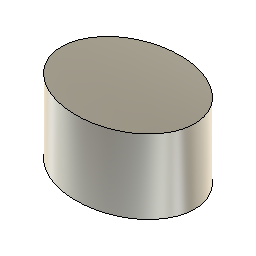
Seed Distribution System v19 (Autodesk Fusion 360 archive; units mm, degrees)
design "Maize Approximation"
Autodesk Fusion 360 part; units mm, degrees
note: some values were not read from the file. Set by a fixed rule: which face or edge a step refers to.
sketch "Sketch1" plane through (0, 0, 0) normal (0, 0, 1) x (1, 0, 0)
  ellipse E0 centre (0, 0) end of major axis (4.5, 0) minor radius 3.5
  line L0 (-4.5, 0) -> (4.5, 0) construction
  line L1 (0, -3.5) -> (0, 3.5) construction
  dimension "d1" = 7
  constraint coincident E0 L0.start
  constraint coincident E0 L0.end
  constraint coincident E0 L1.start
  constraint coincident E0 L1.end
  constraint coincident E0.centre origin
  constraint horizontal L0
extrude "Extrude1" add sketch "Sketch1" along normal blind 5

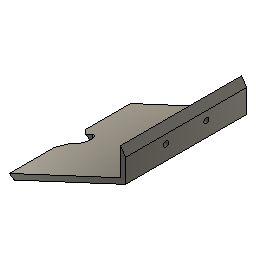
design "H-L1"
Autodesk Fusion 360 part; units mm, degrees
sketch "Sketch1" plane through (0, 0, 0) normal (0, 1, 0) x (1, 0, 0)
  line L0 (0, 0) -> (0, -20)
  line L1 (0, -20) -> (5, -20)
  line L2 (5, -20) -> (5, 0)
  line L3 (0, 0) -> (-107.5153, 50.1352)
  line L4 (-107.5153, 50.1352) -> (-105.4022, 54.6667)
  line L5 (5, 0) -> (5, 3.186)
  line L6 (-105.4022, 54.6667) -> (5, 3.1854)
  line L7 (0, -20) -> (0, -27.5)
  line L8 (0, -27.5) -> (5, -20)
  line L9 (-105.4022, 54.6667) -> (-110.1316, 51.3552)
  line L10 (-105.4022, 54.6667) -> (-105.6539, 54.6667) construction
  line L11 (-110.1316, 51.3552) -> (-107.5153, 50.1352)
  line L12 (0, 0) -> (0, 5.5169) construction
  dimension "d1" = 20
  dimension "d2" = 5
  dimension "d3" = 118.63
  dimension "d4" = 115
  dimension "d5" = 5
  dimension "d7" = 3.186
  dimension "d8" = 7.5
  dimension "d9" = 35
  constraint vertical L0
  constraint coincident L0.start L3.start
  constraint perpendicular L0 L1
  constraint perpendicular L1 L2
  constraint perpendicular L3 L4
  constraint parallel L2 L5
  constraint coincident L5 L6.end
  constraint perpendicular L4 L6
  constraint perpendicular L1 L7
  constraint horizontal L10
  constraint perpendicular L4 L11
  constraint coincident L6 L12.end
  constraint parallel L0 L12
  measures "d1" distance of L0.start L0.end
  measures "d2" distance of L0.end L1.end
  measures "d3" distance of L0.start L3.end
  measures "d4" angle of L0 L3
  measures "d5" distance of L3.end L4.end
  measures "d7" distance of L2.end L5.end
  measures "d8" distance of L0.end L7.end
  measures "d9" angle of L9 L10
extrude "Extrude1" add sketch "Sketch1" along normal blind 120
sketch "Sketch2" plane through (0, 0, 0) normal (-0.422618, 0, 0.906308) x (0, -1, 0)
  line L0 (0, -121.5168) -> (0, 0)
  line L1 (0, 0) -> (-120, 0)
  line L2 (-120, 0) -> (-120, -121.5168)
  line L3 (-120, -121.5168) -> (0, -121.5168)
  line L4 (-60, -121.5168) -> (-60, 0) construction
  line L5 (-60, -121.5168) -> (-52.5, -121.5168)
  line L6 (-52.5, -121.5168) -> (-52.5, -118.6298)
  line L7 (-52.5, -118.6298) -> (-52.5, -105.6298)
  line L8 (-52.5, -105.6298) -> (-60, -105.6298) construction
  circle A0 centre (-60, -105.6298) radius 7.5
  line L9 (-67.5, -105.6298) -> (-67.5, -121.5168)
  dimension "d12" = 7.5
  dimension "d13" = 2.887
  dimension "d14" = 13
  constraint midpoint L3 L4.start
  constraint midpoint L1 L4.end
  constraint perpendicular L4 L5
  constraint perpendicular L3 L6
  constraint parallel L6 L7
  constraint coincident L4 L8.end
  constraint perpendicular L4 L8
  constraint coincident L8.end A0.centre
  constraint coincident L7.end A0
  constraint coincident A0 L9.start
  constraint tangent A0 L9
  constraint perpendicular L3 L9
  measures "d12" distance of L4.start L5.end
  measures "d13" distance of L5.end L6.end
  measures "d14" distance of L6.end L7.end
extrude "Extrude2" cut sketch "Sketch2" against normal blind 5 contours L3 L5 L6 L7 A0 L9 | A0
sketch "Sketch3" plane through (0, 0, 0) normal (-1, 0, 0) x (0, -1, 0)
  line L0 (0, 0) -> (0, 27.5)
  line L1 (0, 27.5) -> (-120, 27.5)
  line L2 (-120, 27.5) -> (-120, 0)
  line L3 (-60, 0) -> (-60, 27.5) construction
  line L4 (-60, 27.5) -> (-60, 11.5) construction
  line L5 (-60, 11.5) -> (-40, 11.5) construction
  circle A0 centre (-40, 11.5) radius 2.6
  circle A1 centre (-80, 11.5) radius 2.6
  line L6 (-120, 0) -> (0, 0)
  dimension "d17" = 16
  dimension "d18" = 20
  dimension "d19" = 5.2
  constraint midpoint L1 L3.end
  constraint perpendicular L1 L4
  constraint perpendicular L0 L5
  constraint coincident L5.end A0.centre
  constraint symmetric L3 A0 A1
  measures "d17" distance of L3.end L4.end
  measures "d18" distance of L4.end L5.end
  measures "d19" diameter of A0
extrude "Extrude3" cut sketch "Sketch3" against normal blind 5 contours A0 | A1
chamfer "Chamfer1" distance 8 angle 45 2 edges at (-107.7669, 67.5, -53.011) (-107.7669, 52.5, -53.011)
equation "d3 = 5.517 mm + 107 mm - 2.887 mm + 9 mm"
equation "d4 = 90 deg + 25 deg"

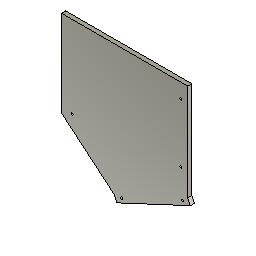
design "H-Left"
Autodesk Fusion 360 part; units mm, degrees
sketch "Sketch1" plane through (0, 0, 0) normal (0, 1, 0) x (1, 0, 0)
  line L0 (0, 0) -> (106.038, -49.4463) construction
  line L1 (0, 0) -> (117, 0) construction
  line L2 (0, 0) -> (-76.6044, -64.2788)
  line L3 (0, 0) -> (-100, 0) construction
  line L4 (-76.6044, -64.2788) -> (-76.6044, -189.2788)
  line L5 (0, 0) -> (106.038, -49.4463)
  line L6 (-76.6044, -64.2788) -> (-71.6044, -64.2788) construction
  line L7 (0, 0) -> (5, 0) construction
  line L8 (0, 0) -> (3.7558, 8.0543)
  line L9 (3.7558, 8.0543) -> (109.7938, -41.3921)
  line L10 (3.7558, 8.0543) -> (119.5357, 8.0543) construction
  line L11 (109.7938, -41.3921) -> (106.038, -49.4463)
  line L12 (3.7558, 8.0543) -> (1.4314, 3.0696) construction
  line L13 (1.4314, 3.0696) -> (10.4944, -1.1566) construction
  circle A0 centre (10.4944, -1.1566) radius 1.6
  line L14 (56.7748, -16.6689) -> (53.019, -24.7232) construction
  circle A1 centre (98.4063, -42.1506) radius 1.6
  line L15 (106.038, -49.4463) -> (106.038, -189.279)
  line L16 (106.038, -189.279) -> (-76.6044, -189.2788)
  line L17 (-76.6044, -64.2788) -> (-58.6287, -72.661) construction
  line L18 (-76.6044, -64.2788) -> (-56.7704, -64.2788) construction
  line L19 (-58.6287, -72.661) -> (-61.6287, -72.661) construction
  line L20 (-61.6287, -72.661) -> (-61.6287, -70.363) construction
  circle A2 centre (-61.6287, -70.363) radius 1.6
  line L21 (-61.6287, -70.363) -> (-61.2829, -70.7751) construction
  line L22 (-61.6287, -70.363) -> (-61.0907, -70.363) construction
  circle A3 centre (-61.2829, -70.7751) radius 1.6
  line L23 (106.038, -189.279) -> (106.038, -168.279) construction
  line L24 (106.038, -168.279) -> (96.038, -168.279) construction
  circle A4 centre (96.038, -168.279) radius 1.6
  line L25 (96.038, -168.279) -> (96.0382, -83.011) construction
  circle A5 centre (96.0382, -83.011) radius 1.6
  dimension "d1" = 117
  dimension "d2" = 25
  dimension "d3" = 100
  dimension "d4" = 40
  dimension "d5" = 125
  dimension "d16" = 8.8869
  dimension "d17" = 25
  dimension "d18" = 117
  dimension "d19" = 5.5
  dimension "d20" = 10
  dimension "d21" = 3.2
  dimension "d25" = 139.8327
  dimension "d26" = 25
  dimension "d27" = 19.834
  dimension "d33" = 3
  dimension "d34" = 2.298
  dimension "d35" = 3.2
  dimension "d38" = 310
  dimension "d39" = 0.538
  dimension "d42" = 3.2
  dimension "d45" = 21
  dimension "d46" = 10
  dimension "d47" = 3.2
  dimension "d48" = 85.268
  dimension "d49" = 3.2
  constraint horizontal L1
  constraint coincident L0.start L1.start
  constraint parallel L1 L3
  constraint vertical L4
  constraint horizontal L6
  constraint horizontal L7
  constraint perpendicular L0 L8
  constraint horizontal L10
  constraint perpendicular L9 L12
  constraint perpendicular L8 L13
  constraint coincident L13.end A0.centre
  constraint midpoint L9 L14.start
  constraint midpoint L5 L14.end
  constraint symmetric A0 L14 A1
  constraint vertical L15
  constraint horizontal L18
  constraint horizontal L19
  constraint perpendicular L19 L20
  constraint coincident L20.end A2.centre
  constraint horizontal L22
  constraint coincident L21.end A3.centre
  constraint perpendicular L16 L23
  constraint perpendicular L23 L24
  constraint coincident L24.end A4.centre
  constraint perpendicular L24 L25
  constraint coincident L25.end A5.centre
  measures "d1" distance of L0.start L0.end
  measures "d2" angle of L0 L1
  measures "d3" distance of L0.start L2.end
  measures "d4" angle of L2 L3
  measures "d5" distance of L2.end L4.end
  measures "d16" distance of L0.start L8.end
  measures "d17" angle of L9 L10
  measures "d18" distance of L8.end L9.end
  measures "d19" distance of L8.end L12.end
  measures "d20" distance of L12.end L13.end
  measures "d21" diameter of A0
  measures "d25" distance of L0.end L15.end
  measures "d26" angle of L17 L18
  measures "d27" distance of L2.end L17.end
  measures "d33" distance of L17.end L19.end
  measures "d34" distance of L19.end L20.end
  measures "d35" diameter of A2
  measures "d39" distance of L20.end L21.end
  measures "d42" diameter of A3
  measures "d45" distance of L15.end L23.end
  measures "d46" distance of L23.end L24.end
  measures "d47" diameter of A4
  measures "d48" distance of L24.end L25.end
  measures "d49" diameter of A5
extrude "Extrude1" add sketch "Sketch1" against normal blind 5 contours L2 L4 L5 L15 L16 | L5 L8 L9 L11 | A0 | A1 | A2 A3 | A2 A3 | A2 A3 | A4 | A5
extrude "Extrude2" cut sketch "Sketch1" against normal blind 5 contours A0 | A1
extrude "Extrude5" cut sketch "Sketch1" against normal blind 5 contours A2 A3 | A2 A3 picked at (-61.7312, -70.2246) picked at (-62.4248, -69.4143)
extrude "Extrude6" add sketch "Sketch1" against normal blind 5 contours A2 A3 | A2 A3 picked at (-61.7312, -70.2246) picked at (-62.4248, -69.4143)
extrude "Extrude7" cut sketch "Sketch1" against normal blind 5 contours A2 A3 | A2 A3 picked at (-61.7312, -70.2246) picked at (-60.3048, -71.8013)
extrude "Extrude8" cut sketch "Sketch1" against normal blind 5 contours A4 | A5
extrude "Extrude9" add 1 faces at (-14.055, -5, 143.0174) along direction (0, -1, 0) blind 1
sketch "Sketch2" plane through (0, -6, 0) normal (0, -1, 0) x (1, 0, 0)
  circle A0 centre (96.0382, 83.011) radius 1.6
  circle A1 centre (96.038, 168.279) radius 1.6
  circle A2 centre (-61.2829, 70.7751) radius 1.6
  circle A3 centre (98.4063, 42.1506) radius 1.6
  circle A4 centre (10.4944, 1.1566) radius 1.6
  line L0 (-76.6044, 64.2788) -> (0, 0)
  line L1 (0, 0) -> (3.7558, -8.0543)
  line L2 (3.7558, -8.0543) -> (109.7938, 41.3921)
  line L3 (109.7938, 41.3921) -> (106.038, 49.4463)
  line L4 (106.038, 49.4463) -> (106.038, 189.279)
  line L5 (106.038, 189.279) -> (-76.6044, 189.2788)
  line L6 (-76.6044, 189.2788) -> (-76.6044, 64.2788)
equation "d16 = 11 mm - 2.11309 mm"
equation "d48 = 86 mm - 0.732 mm"

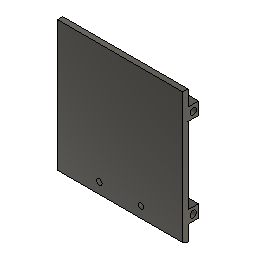
design "H-Front"
Autodesk Fusion 360 part; units mm, degrees
sketch "Sketch1" plane through (0, 0, 0) normal (0, 1, 0) x (1, 0, 0)
  line L0 (0, 0) -> (120, 0)
  line L1 (120, 0) -> (120, -127.268)
  line L2 (120, -127.268) -> (0, -127.268)
  line L3 (0, -127.268) -> (0, 0)
  dimension "d1" = 120
  dimension "d2" = 127.268
  constraint horizontal L0
  constraint vertical L1
  constraint horizontal L2
  constraint vertical L3
  constraint coincident L0.start L3.end
  measures "d1" distance of L0.start L0.end
  measures "d2" distance of L0.start L2.end
extrude "Extrude1" add sketch "Sketch1" along normal blind 5
sketch "Sketch2" plane through (0, 0, 0) normal (-1, 0, 0) x (0, -1, 0)
  line L0 (0, 0) -> (0, 127.268)
  line L1 (0, 127.268) -> (-5, 127.268)
  line L2 (-5, 127.268) -> (-5, 0)
  line L3 (-5, 0) -> (0, 0)
  line L4 (-5, 0) -> (0.0001, 2.3316)
  line L5 (-5, 0) -> (0.517, 0) construction
  line L6 (0, 0) -> (0.0001, 2.3316)
  dimension "d5" = 25
  dimension "d6" = 5.517
  constraint horizontal L5
  constraint coincident L2.end L3.start
  constraint coincident L0.start L3.end
  measures "d5" angle of L4 L5
  measures "d6" distance of L2.end L4.end
extrude "Extrude2" cut sketch "Sketch2" against normal blind 120 contours L0 L3 L4 L6
sketch "Sketch3" plane through (0, 5, 0) normal (0, 1, 0) x (-1, 0, 0)
  line L0 (0, 127.268) -> (-120, 127.268)
  line L1 (-120, 127.268) -> (-120, 0)
  line L2 (-120, 0) -> (0, 0)
  line L3 (0, 0) -> (0, 127.268)
  line L4 (-60, 0) -> (-60, 127.268)
  line L5 (-120, 0) -> (-120, 15) construction
  line L6 (-120, 15) -> (-108, 15)
  line L7 (-108, 15) -> (-108, 27)
  line L8 (-108, 27) -> (-120, 27)
  line L9 (-120, 27) -> (-120, 15)
  line L10 (-120, 63.634) -> (0, 63.634)
  line L11 (0, 27) -> (0, 15)
  line L12 (-12, 27) -> (0, 27)
  line L13 (0, 15) -> (-12, 15)
  line L14 (-12, 15) -> (-12, 27)
  line L15 (-108, 100.268) -> (-120, 100.268)
  line L16 (-120, 100.268) -> (-120, 112.268)
  line L17 (-120, 112.268) -> (-108, 112.268)
  line L18 (-108, 112.268) -> (-108, 100.268)
  line L19 (-12, 112.268) -> (-12, 100.268)
  line L20 (0, 112.268) -> (-12, 112.268)
  line L21 (0, 100.268) -> (0, 112.268)
  line L22 (-12, 100.268) -> (0, 100.268)
  line L23 (-60, 0) -> (-60, 12.6415) construction
  line L24 (-60, 12.6415) -> (-40, 12.6415) construction
  circle A0 centre (-40, 12.6415) radius 2.6
  circle A1 centre (-80, 12.6415) radius 2.6
  dimension "d9" = 15
  dimension "d10" = 12
  dimension "d11" = 12
  dimension "d19" = 12.6415
  dimension "d20" = 20
  dimension "d21" = 5.2
  constraint midpoint L2 L4.start
  constraint midpoint L0 L4.end
  constraint coincident L1.end L2.start
  constraint perpendicular L0 L5
  constraint horizontal L6
  constraint vertical L7
  constraint horizontal L8
  constraint vertical L9
  constraint midpoint L1 L10.start
  constraint midpoint L3 L10.end
  constraint symmetric L4 L5.end L11.end
  constraint symmetric L4 L6.end L13.end
  constraint symmetric L4 L7.end L12.start
  constraint symmetric L4 L8.end L11.start
  constraint symmetric L5.end L10 L16.end
  constraint symmetric L6.end L10 L17.end
  constraint symmetric L7.end L10 L15.start
  constraint symmetric L8.end L10 L15.end
  constraint symmetric L10 L11.start L21.start
  constraint symmetric L10 L11.end L20.start
  constraint symmetric L10 L12.start L19.end
  constraint symmetric L10 L13.end L19.start
  constraint perpendicular L2 L23
  constraint perpendicular L23 L24
  constraint coincident L24.end A0.centre
  constraint symmetric L4 A0 A1
  measures "d9" distance of L1.end L5.end
  measures "d10" distance of L5.end L6.end
  measures "d11" distance of L5.end L8.end
  measures "d19" distance of L4.start L23.end
  measures "d20" distance of L23.end L24.end
  measures "d21" diameter of A0
extrude "Extrude3" add sketch "Sketch3" along normal blind 10 contours L3 L19 L20 L21 L22 | L1 L15 L16 L17 L18 | L1 L6 L7 L8 L9 | L3 L11 L12 L13 L14
sketch "Sketch4" plane through (120, 0, 0) normal (1, 0, 0) x (0, 1, 0)
  line L0 (0, 2.3315) -> (5, 0)
  line L1 (5, 0) -> (5, 15)
  line L2 (5, 15) -> (15, 15)
  line L3 (15, 15) -> (15, 27)
  line L4 (15, 27) -> (5, 27)
  line L5 (5, 27) -> (5, 100.268)
  line L6 (5, 100.268) -> (15, 100.268)
  line L7 (15, 100.268) -> (15, 112.268)
  line L8 (15, 112.268) -> (5, 112.268)
  line L9 (5, 112.268) -> (5, 127.268)
  line L10 (5, 127.268) -> (0, 127.268)
  line L11 (0, 127.268) -> (0, 2.3315)
  line L12 (5, 27) -> (15, 15) construction
  line L13 (5, 15) -> (15, 27) construction
  circle A0 centre (10, 21) radius 3.1
  line L14 (5, 63.634) -> (0, 63.634) construction
  circle A1 centre (10, 106.268) radius 3.1
  dimension "d14" = 6.2
  constraint coincident L4.end L5.start
  constraint coincident L2.end L3.start
  constraint coincident L1.end L2.start
  constraint coincident L3.end L4.start
  constraint midpoint L12 A0.centre
  constraint midpoint L5 L14.start
  constraint coincident L11 L14.end
  constraint perpendicular L11 L14
  constraint symmetric A0 L14 A1
  measures "d14" diameter of A0
extrude "Extrude4" cut sketch "Sketch4" against normal blind 7 contours A0 | A1
ref_plane "WorkPlane1" through (60, 10, 106.268) normal (1, 0, 0) x (0, 0, -1)
mirror "Mirror1" about plane through (60, 10, 106.268) normal (1, 0, 0) of "Extrude4"
extrude "Extrude5" cut sketch "Sketch3" against normal blind 5 contours A0 | A1
equation "d2 = 139.8 mm - 5 mm - 7.332 mm - 0.2 mm"
equation "d19 = 11.5 mm + 0.1415 mm + 1 mm"

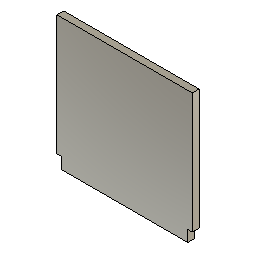
design "H-Back"
Autodesk Fusion 360 part; units mm, degrees
sketch "Sketch1" plane through (0, 0, 0) normal (0, 1, 0) x (1, 0, 0)
  line L0 (0, 0) -> (120, 0)
  line L1 (120, 0) -> (120, -116.886)
  line L2 (120, -116.886) -> (0, -116.886)
  line L3 (0, -116.886) -> (0, 0)
  line L4 (0, 0) -> (0, -10) construction
  line L5 (0, -10) -> (4, -10)
  line L6 (4, -10) -> (4, 0)
  line L7 (60, 0) -> (60, -116.886) construction
  line L8 (120, -10) -> (116, -10)
  line L9 (116, -10) -> (116, 0)
  dimension "d1" = 120
  dimension "d2" = 116.886
  dimension "d3" = 10
  dimension "d4" = 4
  constraint horizontal L0
  constraint vertical L1
  constraint horizontal L2
  constraint vertical L3
  constraint coincident L0.start L3.end
  constraint perpendicular L0 L4
  constraint perpendicular L4 L5
  constraint coincident L0 L6.end
  constraint perpendicular L0 L6
  constraint midpoint L0 L7.start
  constraint midpoint L2 L7.end
  constraint symmetric L4.end L7 L8.start
  constraint symmetric L5.end L7 L8.end
  constraint symmetric L6.end L7 L9.end
  measures "d1" distance of L0.start L0.end
  measures "d2" distance of L0.start L2.end
  measures "d3" distance of L0.start L4.end
  measures "d4" distance of L4.end L5.end
extrude "Extrude1" add sketch "Sketch1" along normal blind 5 contours L0 L1 L2 L3 L5 L6 L8 L9
extrude "Extrude2" add 1 faces at (41.3333, 5, 81.2573) along direction (0, 1, 0) blind 1
sketch "Sketch2" plane through (0, 0, 0) normal (0, -1, 0) x (1, 0, 0)
  line L0 (116, 10) -> (120, 10)
  line L1 (120, 10) -> (120, 116.886)
  line L2 (120, 116.886) -> (0, 116.886)
  line L3 (0, 116.886) -> (0, 10)
  line L4 (0, 10) -> (4, 10)
  line L5 (4, 10) -> (4, 0)
  line L6 (4, 0) -> (116, 0)
  line L7 (116, 0) -> (116, 10)

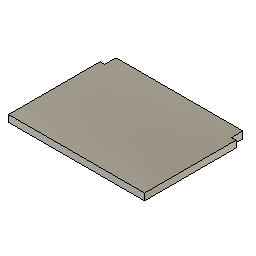
design "H-Bottom"
Autodesk Fusion 360 part; units mm, degrees
sketch "Sketch1" plane through (0, 0, 0) normal (0, 0, 1) x (1, 0, 0)
  line L0 (0, 0) -> (120, 0)
  line L1 (120, 0) -> (120, 90.821)
  line L2 (120, 90.821) -> (0, 90.821)
  line L3 (0, 90.821) -> (0, 0)
  line L4 (4, 90.821) -> (4, 80.821)
  line L5 (4, 80.821) -> (0, 80.821)
  line L6 (60, 0) -> (60, 90.821) construction
  line L7 (116, 80.821) -> (120, 80.821)
  line L8 (116, 90.821) -> (116, 80.821)
  dimension "d1" = 120
  dimension "d2" = 90.821
  dimension "d8" = 4
  dimension "d9" = 4
  dimension "d10" = 10
  dimension "d11" = 10
  constraint horizontal L0
  constraint vertical L1
  constraint horizontal L2
  constraint vertical L3
  constraint coincident L0.start L3.end
  constraint vertical L4
  constraint horizontal L5
  constraint midpoint L0 L6.start
  constraint midpoint L2 L6.end
  constraint symmetric L4.start L6 L8.start
  constraint symmetric L4.end L6 L7.start
  constraint symmetric L5.end L6 L7.end
  measures "d1" distance of L0.start L0.end
  measures "d2" distance of L0.start L2.end
  measures "d8" distance of L4.end L5.end
  measures "d9" distance of L2.end L4.start
  measures "d10" distance of L4.start L4.end
  measures "d11" distance of L2.end L5.end
extrude "Extrude1" add sketch "Sketch1" along normal blind 5
extrude "Extrude2" cut sketch "Sketch1" along normal blind 5 contours L2 L3 L4 L5 | L1 L2 L7 L8
move_face "OffsetFaces1" offset 1 1 faces at (78.6667, 26.9403, 0)
sketch "Sketch2" plane through (0, 0, 5) normal (0, 0, 1) x (-1, 0, 0)
  line L0 (-4, -90.821) -> (-4, -80.821)
  line L1 (-4, -80.821) -> (0, -80.821)
  line L2 (0, -80.821) -> (0, 0)
  line L3 (0, 0) -> (-120, 0)
  line L4 (-120, 0) -> (-120, -80.821)
  line L5 (-120, -80.821) -> (-116, -80.821)
  line L6 (-116, -80.821) -> (-116, -90.821)
  line L7 (-116, -90.821) -> (-4, -90.821)
equation "d2 = 90 mm + 0.821 mm"

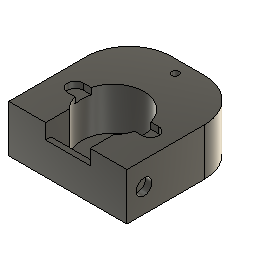
design "Stepper Housing"
Autodesk Fusion 360 part; units mm, degrees
sketch "Sketch1" plane through (0, 0, 0) normal (0, 0, 1) x (1, 0, 0)
  circle A0 centre (0, 0) radius 14.4
  line L0 (-10.3615, -10) -> (10.3615, -10)
  line L1 (0, -10) -> (0, 0) construction
  line L2 (0, 0) -> (17.5, 0) construction
  circle A1 centre (17.5, 0) radius 2.25
  line L3 (-10.3615, -10) -> (-10.3615, -17.5)
  circle A2 centre (-17.5, 0) radius 2.25
  line L4 (10.3615, -10) -> (10.3615, -17.5)
  line L5 (-10.3615, -17.5) -> (-21.3615, -17.5)
  line L6 (-21.3615, -17.5) -> (-21.3615, 17.5)
  line L7 (-21.3615, 17.5) -> (0, 17.5)
  line L8 (10.3615, -17.5) -> (21.3615, -17.5)
  line L9 (21.3615, -17.5) -> (21.3615, 17.5)
  line L10 (21.3615, 17.5) -> (0, 17.5)
  line L11 (-10.3615, -17.5) -> (10.3615, -17.5)
  line L12 (0, 0) -> (0, 8) construction
  circle A3 centre (0, 8) radius 50 construction
  dimension "d1" = 28.8
  dimension "d2" = 10
  dimension "d3" = 17.5
  dimension "d4" = 4.5
  dimension "d5" = 7.5
  dimension "d7" = 7.5
  dimension "d8" = 11
  dimension "d9" = 35
  dimension "d16" = 8
  dimension "d17" = 100
  constraint coincident A0.centre L1.end
  constraint coincident A0 L0.start
  constraint coincident A0 L0.end
  constraint horizontal L0
  constraint midpoint L0 L1.start
  constraint perpendicular L1 L2
  constraint coincident L2.end A1.centre
  constraint perpendicular L0 L3
  constraint symmetric L1 A1 A2
  constraint perpendicular L0 L4
  constraint perpendicular L3 L5
  constraint perpendicular L5 L6
  constraint perpendicular L6 L7
  constraint symmetric L1 L3.end L4.end
  constraint symmetric L1 L5.end L8.end
  constraint symmetric L1 L6.end L9.end
  constraint symmetric L1 L7.end L10.end
  constraint perpendicular L2 L12
  constraint coincident L12.end A3.centre
  measures "d1" diameter of A0
  measures "d2" distance of L1.start A0.centre
  measures "d3" distance of A0.centre L2.end
  measures "d4" diameter of A1
  measures "d5" distance of L0.start L3.end
  measures "d7" distance of L0.end L4.end
  measures "d8" distance of L3.end L5.end
  measures "d9" distance of L5.end L6.end
  measures "d16" distance of A0.centre L12.end
  measures "d17" diameter of A3
extrude "Extrude1" add sketch "Sketch1" along normal blind 18 contours A0 L3 L4 L5 L6 L7 L8 L9 L10
extrude "Extrude2" add sketch "Sketch1" along normal blind 12 contours A1 | A2
extrude "Extrude3" add sketch "Sketch1" against normal blind 3 contours A0 L0 | A0 L3 L4 L5 L6 L7 L8 L9 L10 | A0 L0 | A0 L3 L4 L11 | A1 | A2
sketch "Sketch2" plane through (0, 0, -3) normal (0, 0, -1) x (1, 0, 0)
  line L0 (21.3615, 17.5) -> (-21.3615, 17.5)
  line L1 (-21.3615, 17.5) -> (-21.3615, -17.5)
  line L2 (-21.3615, -17.5) -> (21.3615, -17.5)
  line L3 (21.3615, -17.5) -> (21.3615, 17.5)
  line L4 (21.3615, 17.5) -> (-21.3615, 17.5)
  line L5 (-21.3615, 17.5) -> (-21.3615, 21)
  line L6 (-21.3615, 21) -> (21.3615, 21)
  line L7 (21.3615, 21) -> (21.3615, 17.5)
  line L8 (-21.3615, 17.5) -> (-10.3615, 17.5) construction
  line L9 (-10.3615, 17.5) -> (-10.3615, 21)
  line L10 (0, 0) -> (0, 17.5) construction
  line L11 (10.3615, 17.5) -> (10.3615, 21)
  line L12 (-21.3615, 21) -> (-27.5, 21)
  line L13 (-27.5, 21) -> (-27.5, -35)
  line L14 (-27.5, -35) -> (0, -35)
  line L15 (21.3615, 21) -> (27.5, 21)
  line L16 (27.5, 21) -> (27.5, -35)
  line L17 (27.5, -35) -> (0, -35)
  line L18 (-10.3615, 17.5) -> (10.3615, 17.5)
  line L19 (10.3615, 17.5) -> (10.3615, 18.5)
  line L20 (10.3615, 18.5) -> (-10.3615, 18.5)
  line L21 (-10.3615, 18.5) -> (-10.3615, 17.5)
  dimension "d18" = 3.5
  dimension "d19" = 42.7229
  dimension "d20" = 11
  dimension "d25" = 6.1385
  dimension "d26" = 56
  dimension "d49" = 1
  dimension "d50" = 20.7229
  constraint horizontal L4
  constraint vertical L5
  constraint horizontal L6
  constraint vertical L7
  constraint coincident L0.start L3.end
  constraint perpendicular L1 L8
  constraint coincident L6 L9.end
  constraint perpendicular L6 L9
  constraint coincident L10.start origin
  constraint midpoint L0 L10.end
  constraint symmetric L8.end L10 L11.start
  constraint symmetric L9.end L10 L11.end
  constraint perpendicular L5 L12
  constraint perpendicular L12 L13
  constraint perpendicular L13 L14
  constraint symmetric L5.end L10 L6.end
  constraint symmetric L10 L12.end L15.end
  constraint symmetric L10 L13.end L16.end
  constraint symmetric L10 L14.end L17.end
  constraint horizontal L18
  constraint vertical L19
  constraint horizontal L20
  constraint vertical L21
  measures "d18" distance of L0.start L6.end
  measures "d19" distance of L5.end L6.end
  measures "d20" distance of L0.end L8.end
  measures "d25" distance of L5.end L12.end
  measures "d26" distance of L12.end L13.end
  measures "d49" distance of L8.end L20.end
  measures "d50" distance of L19.end L20.end
extrude "Extrude4" add sketch "Sketch2" against normal blind 21 contours L0 L4 L6 L7 L11 L19 | L0 L4 L5 L6 L9 L21
extrude "Extrude5" add sketch "Sketch2" against normal blind 10 contours L0 L4 L9 L11 L18 L19 L20 L21 | L6 L9 L11 L20
extrude "Extrude6" add sketch "Sketch2" against normal blind 21 contours L1 L2 L3 L5 L7 L12 L13 L14 L15 L16 L17
sketch "Sketch3" plane through (0, 0, 18) normal (0, 0, 1) x (-1, 0, 0)
  circle A0 centre (17.5, 0) radius 2.25
  circle A1 centre (-17.5, 0) radius 2.25
  line L0 (-10.3615, 10) -> (-10.3615, 21)
  line L1 (-10.3615, 21) -> (-27.5, 21)
  line L2 (-27.5, 21) -> (-27.5, -35)
  line L3 (-27.5, -35) -> (27.5, -35)
  line L4 (27.5, -35) -> (27.5, 21)
  line L5 (27.5, 21) -> (10.3615, 21)
  line L6 (10.3615, 21) -> (10.3615, 10)
  arc A2 (-10.3615, 10) -> (10.3615, 10) centre (0, 0) ccw
  circle A3 centre (17.5, 0) radius 4.5
  line L7 (17.5, 0) -> (17.5, -4.5) construction
  line L8 (17.5, -4.5) -> (13.6788, -4.5)
  line L9 (17.5, 0) -> (17.5, 4.5) construction
  line L10 (17.5, 4.5) -> (13.6788, 4.5)
  line L11 (0, 0) -> (0, -14.4) construction
  line L12 (-17.5, -4.5) -> (-13.6788, -4.5)
  circle A4 centre (-17.5, 0) radius 4.5
  line L13 (-17.5, 4.5) -> (-13.6788, 4.5)
  line L14 (0, -14.4) -> (0, -29.05) construction
  circle A5 centre (0, -29.05) radius 1.65
  circle A6 centre (17.5, 0) radius 2.25 construction
  circle A7 centre (-17.5, 0) radius 2.25 construction
  dimension "d29" = 9
  dimension "d30" = 4.5
  dimension "d31" = 4.5
  dimension "d32" = 14.65
  dimension "d33" = 3.3
  dimension "d34" = 4.5
  dimension "d35" = 4.5
  constraint concentric A0 A3
  constraint coincident A0.centre A3.centre
  constraint vertical L7
  constraint coincident A2 L8.end
  constraint tangent A3 L8
  constraint perpendicular L7 L8
  constraint perpendicular L8 L9
  constraint coincident A2 L10.end
  constraint tangent A3 L10
  constraint perpendicular L9 L10
  constraint coincident A2.centre L11.start
  constraint midpoint A2 L11.end
  constraint symmetric A3 L11 A4
  constraint symmetric L7.end L11 L12.start
  constraint symmetric L8.end L11 L12.end
  constraint symmetric L9.end L11 L13.start
  constraint symmetric L10.end L11 L13.end
  constraint perpendicular L3 L14
  constraint coincident L14.end A5.centre
  constraint concentric A4 A7
  measures "d29" diameter of A3
  measures "d30" distance of A0.centre L7.end
  measures "d31" distance of A0.centre L9.end
  measures "d32" distance of L11.end L14.end
  measures "d33" diameter of A5
  measures "d34" diameter of A6
  measures "d35" diameter of A7
extrude "Extrude7" add sketch "Sketch3" along normal blind 1 contours L0 L1 L2 L3 L4 L5 L6 A2 A3 L8 L10 L12 A4 L13
extrude "Extrude8" cut 2 faces at (-16.1057, 3.108, 18) (16.1057, -3.108, 18) along direction (0, 0, -1) blind 3
extrude "Extrude9" add 2 faces at (-16.9203, 0.5864, 12) (17.9871, 0.6495, 12) along direction (0, 0, 1) blind 3
sketch "Sketch4" plane through (0, 0, -3) normal (0, 0, -1) x (1, 0, 0)
  line L0 (27.5, 21) -> (-27.5, 21)
  line L1 (-27.5, 21) -> (-27.5, -35)
  line L2 (-27.5, -35) -> (27.5, -35)
  line L3 (27.5, -35) -> (27.5, 21)
  line L4 (0, -35) -> (8, -35) construction
  line L5 (8, -35) -> (-8, -35)
  line L6 (-8, -35) -> (-8, -23)
  line L7 (-8, -23) -> (8, -23)
  line L8 (8, -23) -> (8, -35)
  dimension "d42" = 8
  dimension "d43" = 16
  dimension "d44" = 12
  constraint midpoint L2 L4.start
  constraint parallel L2 L4
  constraint horizontal L5
  constraint vertical L6
  constraint horizontal L7
  constraint vertical L8
  measures "d42" distance of L4.start L4.end
  measures "d43" distance of L4.end L5.end
  measures "d44" distance of L4.end L7.end
extrude "Extrude10" cut 1 faces at (0.4955, 28.8114, 18) along direction (0, 0, -1) blind 2
extrude "Extrude11" cut sketch "Sketch4" against normal blind 19 contours L2 L5 L6 L7 L8
extrude "Extrude12" cut sketch "Sketch2" against normal blind 10 contours L0 L4 L9 L11 L18 L19 L20 L21
extrude "Extrude13" add sketch "Sketch2" against normal blind 3 contours L0 L4 L9 L11 L18 L19 L20 L21
extrude "Extrude14" add 1 faces at (3.4538, -19.3333, 7) along direction (0, 0, 1) blind 5
sketch "Sketch5" plane through (-27.5, 0, 0) normal (-1, 0, 0) x (0, -1, 0)
  line L0 (-35, -3) -> (21, -3)
  line L1 (21, -3) -> (21, 19)
  line L2 (21, 19) -> (-35, 19)
  line L3 (-35, 19) -> (-35, -3)
  line L4 (21, 8) -> (13, 8) construction
  circle A0 centre (13, 8) radius 3.65
  dimension "d57" = 8
  dimension "d58" = 7.3
  constraint midpoint L1 L4.start
  constraint perpendicular L1 L4
  constraint coincident L4.end A0.centre
  measures "d57" distance of L4.start L4.end
  measures "d58" diameter of A0
extrude "Extrude15" cut sketch "Sketch5" against normal blind 3 contours A0
mirror "Mirror1" about plane through (0, 0, 0) normal (1, 0, 0) of "Extrude15"
extrude "Extrude16" add 2 faces at (-16.9098, 0.1121, 15) (16.9098, -0.1121, 15) along direction (0, 0, 1) blind 1.05
move_face "OffsetFaces1" offset -0.75 1 faces at (3.5823, 5.2736, 0)
move_face "OffsetFaces2" offset 0.75 4 faces at (14.9525, 4.5, 17.6833) (19.248, -4.1466, 18.6667) (19.248, -4.1466, 16.7) (14.9525, -4.5, 17.6833)
move_face "OffsetFaces3" offset 0.75 4 faces at (-14.9525, 4.5, 17.6833) (-18.6104, 4.3608, 18.3333) (-18.6104, 4.3608, 16.7) (-14.9525, -4.5, 17.6833)
fillet "Fillet1" radius 20 2 edges at (27.5, 35, 8) (-27.5, 35, 8)
equation "d3 = ( 35 / 2 ) * 1 mm"
equation "d25 = ( ( 55 - 42.723 ) / 2 ) * 1 mm"
equation "d32 = ( 3.3 / 2 ) * 1 mm + 13 mm"
equation "d63 = 2 mm - 0.95 mm"

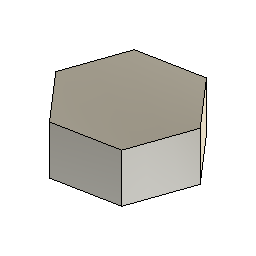
design "M4 Nut Approximation"
Autodesk Fusion 360 part; units mm, degrees
sketch "Sketch1" plane through (0, 0, 0) normal (0, 0, 1) x (1, 0, 0)
  circle A0 centre (0, 0) radius 4
  line L0 (2.618, -3.0243) -> (3.9281, 0.7551)
  line L1 (3.9281, 0.7551) -> (1.3101, 3.7794)
  line L2 (1.3101, 3.7794) -> (-2.618, 3.0243)
  line L3 (-2.618, 3.0243) -> (-3.9281, -0.7551)
  line L4 (-3.9281, -0.7551) -> (-1.3101, -3.7794)
  line L5 (-1.3101, -3.7794) -> (2.618, -3.0243)
  dimension "d1" = 8
  constraint coincident A0.centre origin
  constraint coincident A0 L0.start
  measures "d1" diameter of A0
extrude "Extrude1" add sketch "Sketch1" along normal blind 3.15 contours L0 L1 L2 L3 L4 L5

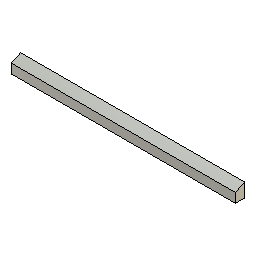
design "H-Front-L1"
Autodesk Fusion 360 part; units mm, degrees
sketch "Sketch1" plane through (0, 0, 0) normal (0, 1, 0) x (1, 0, 0)
  line L0 (0, 0) -> (120, 0)
  line L1 (120, 0) -> (120, -5)
  line L2 (120, -5) -> (0, -5)
  line L3 (0, -5) -> (0, 0)
  dimension "d1" = 120
  dimension "d2" = 5
  constraint horizontal L0
  constraint vertical L1
  constraint horizontal L2
  constraint vertical L3
  constraint coincident L0.start L3.end
  measures "d1" distance of L0.start L0.end
  measures "d2" distance of L0.start L2.end
extrude "Extrude1" add sketch "Sketch1" along normal blind 5
sketch "Sketch2" plane through (120, 0, 0) normal (1, 0, 0) x (0, 1, 0)
  line L0 (0, 5) -> (0, 0)
  line L1 (0, 0) -> (5, 0)
  line L2 (5, 0) -> (5, 5)
  line L3 (5, 5) -> (0, 5)
  line L4 (5, 5) -> (5, 20) construction
  line L5 (0, 5) -> (9.331, 9.3511) construction
  line L6 (5, 5) -> (5, 7.3315)
  line L7 (0, 5) -> (5, 7.3315)
  dimension "d5" = 115
  constraint coincident L2.end L3.start
  constraint perpendicular L3 L4
  constraint coincident L0.start L3.end
  constraint coincident L5 L6.end
  constraint coincident L4 L6.end
  measures "d5" angle of L4 L5
extrude "Extrude2" add sketch "Sketch2" against normal blind 120 contours L3 L6 L7
